Autodesk Inventor part; units mm, degrees
(part 2 of 5)
sketch "Sketch4" plane through (0, 0, 3) normal (0, 0, 1) x (1, 0, 0)
  line L0 (57.5, 215) -> (-78, 215) projected
  line L1 (-78, 215) -> (-78, 46.0635) projected
  line L2 (-78, 46.0635) -> (-75, 46.0635) projected
  line L3 (-75, 46.0635) -> (-75, 40.8932) projected
  line L4 (-75, 40.8932) -> (-78, 40.8932) projected
  line L5 (-78, 40.8932) -> (-78, 30.6062) projected
  line L6 (-78, 30.6062) -> (-75, 30.6062) projected
  line L7 (-75, 30.6062) -> (-75, 20.5478) projected
  line L8 (-75, 20.5478) -> (-78, 20.5478) projected
  line L9 (-78, 20.5478) -> (-78, 10.2608) projected
  line L10 (-78, 10.2608) -> (-75, 10.2608) projected
  line L11 (-75, 10.2608) -> (-75, -0.1068) projected
  line L12 (-75, -0.1068) -> (-78, -0.1068) projected
  line L13 (-78, -0.1068) -> (-78, -10.3938) projected
  line L14 (-78, -10.3938) -> (-75, -10.3938) projected
  line L15 (-75, -10.3938) -> (-75, -20.4522) projected
  line L16 (-75, -20.4522) -> (-78, -20.4522) projected
  line L17 (-78, -20.4522) -> (-78, -30.7392) projected
  line L18 (-78, -30.7392) -> (-75, -30.7392) projected
  line L19 (-75, -30.7392) -> (-75, -41.1068) projected
  line L20 (-75, -41.1068) -> (-78, -41.1068) projected
  line L21 (-78, -41.1068) -> (-78, -51.3938) projected
  line L22 (-78, -51.3938) -> (-75, -51.3938) projected
  line L23 (-75, -51.3938) -> (-75, -61.4522) projected
  line L24 (-75, -61.4522) -> (-78, -61.4522) projected
  line L25 (-78, -61.4522) -> (-78, -71.7392) projected
  line L26 (-78, -71.7392) -> (-75, -71.7392) projected
  line L27 (-75, -71.7392) -> (-75, -82.1068) projected
  line L28 (-75, -82.1068) -> (-78, -82.1068) projected
  line L29 (-78, -82.1068) -> (-78, -92.3938) projected
  line L30 (-78, -92.3938) -> (-75, -92.3938) projected
  line L31 (-75, -92.3938) -> (-75, -102.4522) projected
  line L32 (-75, -102.4522) -> (-78, -102.4522) projected
  line L33 (-78, -102.4522) -> (-78, -130) projected
  line L34 (-78, -130) -> (-55.8933, -130) projected
  line L35 (-55.8933, -130) -> (-55.8933, -135) projected
  line L36 (-55.8933, -135) -> (-25.3933, -135) projected
  line L37 (-25.3933, -135) -> (-25.3933, -147.5) projected
  line L38 (-25.3933, -147.5) -> (23.6067, -147.5) projected
  line L39 (23.6067, -147.5) -> (23.6067, -135) projected
  line L40 (23.6067, -135) -> (54.1067, -135) projected
  line L41 (54.1067, -135) -> (54.1067, -130) projected
  line L42 (54.1067, -130) -> (75, -130) projected
  line L43 (75, -130) -> (75, -111.1237) projected
  arc A0 (75, -111.1237) -> (74, -110.1237) centre (74, -111.1237) ccw projected
  line L44 (74, -110.1237) -> (64.4142, -110.1237) projected
  arc A1 (64.4142, -110.1237) -> (63.7071, -110.4166) centre (64.4142, -111.1237) ccw projected
  line L45 (63.7071, -110.4166) -> (59.2929, -114.8308) projected
  arc A2 (58.5858, -115.1237) -> (59.2929, -114.8308) centre (58.5858, -114.1237) ccw projected
  line L46 (58.5858, -115.1237) -> (43.2196, -115.1237) projected
  arc A3 (42.2196, -114.1237) -> (43.2196, -115.1237) centre (43.2196, -114.1237) ccw projected
  line L47 (42.2196, -114.1237) -> (42.2196, -104.6674) projected
  arc A4 (42.2196, -104.6674) -> (40.773, -102.7455) centre (40.2196, -104.6674) ccw projected
  arc A5 (39.7673, -102.1811) -> (40.773, -102.7455) centre (41.4696, -100.3262) ccw projected
  arc A6 (39.1196, -100.7076) -> (39.7673, -102.1811) centre (41.1196, -100.7076) ccw projected
  line L48 (39.1196, -100.7076) -> (39.1196, -95.7515) projected
  arc A7 (39.7673, -94.2779) -> (39.1196, -95.7515) centre (41.1196, -95.7515) ccw projected
  arc A8 (39.937, -94.1354) -> (39.7673, -94.2779) centre (41.4696, -96.1328) ccw projected
  arc A9 (39.937, -94.1354) -> (40.7196, -92.5486) centre (38.7196, -92.5486) ccw projected
  line L49 (40.7196, -92.5486) -> (40.7196, -83.4104) projected
  arc A10 (40.7196, -83.4104) -> (39.937, -81.8236) centre (38.7196, -83.4104) ccw projected
  arc A11 (39.7673, -81.6811) -> (39.937, -81.8236) centre (41.4696, -79.8262) ccw projected
  arc A12 (39.1196, -80.2076) -> (39.7673, -81.6811) centre (41.1196, -80.2076) ccw projected
  line L50 (39.1196, -80.2076) -> (39.1196, -75.2515) projected
  arc A13 (39.7673, -73.7779) -> (39.1196, -75.2515) centre (41.1196, -75.2515) ccw projected
  arc A14 (39.937, -73.6354) -> (39.7673, -73.7779) centre (41.4696, -75.6328) ccw projected
  arc A15 (39.937, -73.6354) -> (40.7196, -72.0486) centre (38.7196, -72.0486) ccw projected
  line L51 (40.7196, -72.0486) -> (40.7196, -62.9104) projected
  arc A16 (40.7196, -62.9104) -> (39.937, -61.3236) centre (38.7196, -62.9104) ccw projected
  arc A17 (39.7673, -61.1811) -> (39.937, -61.3236) centre (41.4696, -59.3262) ccw projected
  arc A18 (39.1196, -59.7076) -> (39.7673, -61.1811) centre (41.1196, -59.7076) ccw projected
  line L52 (39.1196, -59.7076) -> (39.1196, -54.7515) projected
  arc A19 (39.7673, -53.2779) -> (39.1196, -54.7515) centre (41.1196, -54.7515) ccw projected
  arc A20 (39.937, -53.1354) -> (39.7673, -53.2779) centre (41.4696, -55.1328) ccw projected
  arc A21 (39.937, -53.1354) -> (40.7196, -51.5486) centre (38.7196, -51.5486) ccw projected
  line L53 (40.7196, -51.5486) -> (40.7196, -42.4104) projected
  arc A22 (40.7196, -42.4104) -> (39.937, -40.8236) centre (38.7196, -42.4104) ccw projected
  arc A23 (39.7673, -40.6811) -> (39.937, -40.8236) centre (41.4696, -38.8262) ccw projected
  arc A24 (39.1196, -39.2076) -> (39.7673, -40.6811) centre (41.1196, -39.2076) ccw projected
  line L54 (39.1196, -39.2076) -> (39.1196, -34.2515) projected
  arc A25 (39.7673, -32.7779) -> (39.1196, -34.2515) centre (41.1196, -34.2515) ccw projected
  arc A26 (39.937, -32.6354) -> (39.7673, -32.7779) centre (41.4696, -34.6328) ccw projected
  arc A27 (39.937, -32.6354) -> (40.7196, -31.0486) centre (38.7196, -31.0486) ccw projected
  line L55 (40.7196, -31.0486) -> (40.7196, -21.9104) projected
  arc A28 (40.7196, -21.9104) -> (39.937, -20.3236) centre (38.7196, -21.9104) ccw projected
  arc A29 (39.7673, -20.1811) -> (39.937, -20.3236) centre (41.4696, -18.3262) ccw projected
  arc A30 (39.1196, -18.7076) -> (39.7673, -20.1811) centre (41.1196, -18.7076) ccw projected
  line L56 (39.1196, -18.7076) -> (39.1196, -13.7515) projected
  arc A31 (39.7673, -12.2779) -> (39.1196, -13.7515) centre (41.1196, -13.7515) ccw projected
  arc A32 (39.937, -12.1354) -> (39.7673, -12.2779) centre (41.4696, -14.1328) ccw projected
  arc A33 (39.937, -12.1354) -> (40.7196, -10.5486) centre (38.7196, -10.5486) ccw projected
  line L57 (40.7196, -10.5486) -> (40.7196, -1.4104) projected
  arc A34 (40.7196, -1.4104) -> (39.937, 0.1764) centre (38.7196, -1.4104) ccw projected
  arc A35 (39.7673, 0.3189) -> (39.937, 0.1764) centre (41.4696, 2.1738) ccw projected
  arc A36 (39.1196, 1.7924) -> (39.7673, 0.3189) centre (41.1196, 1.7924) ccw projected
  line L58 (39.1196, 1.7924) -> (39.1196, 6.7485) projected
  arc A37 (39.7673, 8.2221) -> (39.1196, 6.7485) centre (41.1196, 6.7485) ccw projected
  arc A38 (39.937, 8.3646) -> (39.7673, 8.2221) centre (41.4696, 6.3672) ccw projected
  arc A39 (39.937, 8.3646) -> (40.7196, 9.9514) centre (38.7196, 9.9514) ccw projected
  line L59 (40.7196, 9.9514) -> (40.7196, 19.0896) projected
  arc A40 (40.7196, 19.0896) -> (39.937, 20.6764) centre (38.7196, 19.0896) ccw projected
  arc A41 (39.7673, 20.8189) -> (39.937, 20.6764) centre (41.4696, 22.6738) ccw projected
  arc A42 (39.1196, 22.2924) -> (39.7673, 20.8189) centre (41.1196, 22.2924) ccw projected
  line L60 (39.1196, 22.2924) -> (39.1196, 27.2485) projected
  arc A43 (39.7673, 28.7221) -> (39.1196, 27.2485) centre (41.1196, 27.2485) ccw projected
  arc A44 (39.937, 28.8646) -> (39.7673, 28.7221) centre (41.4696, 26.8672) ccw projected
  arc A45 (39.937, 28.8646) -> (40.7196, 30.4514) centre (38.7196, 30.4514) ccw projected
  line L61 (40.7196, 30.4514) -> (40.7196, 39.5896) projected
  arc A46 (40.7196, 39.5896) -> (39.937, 41.1764) centre (38.7196, 39.5896) ccw projected
  arc A47 (39.7673, 41.3189) -> (39.937, 41.1764) centre (41.4696, 43.1738) ccw projected
  arc A48 (39.1196, 42.7924) -> (39.7673, 41.3189) centre (41.1196, 42.7924) ccw projected
  line L62 (39.1196, 42.7924) -> (39.1196, 47.7485) projected
  arc A49 (39.7673, 49.2221) -> (39.1196, 47.7485) centre (41.1196, 47.7485) ccw projected
  arc A50 (43.3362, 49.0566) -> (39.7673, 49.2221) centre (41.4696, 47.3672) ccw projected
  arc A51 (43.3362, 49.0566) -> (44.819, 48.3987) centre (44.819, 50.3987) ccw projected
  line L63 (44.819, 48.3987) -> (75, 48.3987) projected
  line L64 (75, 48.3987) -> (75, 184.5) projected
  line L65 (75, 184.5) -> (57.5, 184.5) projected
  line L66 (57.5, 184.5) -> (57.5, 215) projected
  line L67 (-69.3194, 50.0635) -> (-69.3194, 207.0635) projected
  arc A52 (-68.3194, 208.0635) -> (-69.3194, 207.0635) centre (-68.3194, 207.0635) ccw projected
  line L68 (-68.3194, 208.0635) -> (-25.6194, 208.0635) projected
  arc A53 (-24.6194, 207.0635) -> (-25.6194, 208.0635) centre (-25.6194, 207.0635) ccw projected
  line L69 (-24.6194, 207.0635) -> (-24.6194, 50.0635) projected
  arc A54 (-25.6194, 49.0635) -> (-24.6194, 50.0635) centre (-25.6194, 50.0635) ccw projected
  line L70 (-25.6194, 49.0635) -> (-68.3194, 49.0635) projected
  arc A55 (-69.3194, 50.0635) -> (-68.3194, 49.0635) centre (-68.3194, 50.0635) ccw projected
  arc A56 (-6.9692, 137.8876) -> (4.019, 134.5987) centre (4.019, 154.5987) ccw projected
  arc A57 (-13.8416, 143.5179) -> (-6.9692, 137.8876) centre (16.3806, 173.3987) ccw projected
  arc A58 (-19.6194, 157.5794) -> (-13.8416, 143.5179) centre (0.3806, 157.5794) ccw projected
  line L71 (-19.6194, 157.5794) -> (-19.6194, 189.218) projected
  arc A59 (-13.8416, 203.2796) -> (-19.6194, 189.218) centre (0.3806, 189.218) ccw projected
  arc A60 (-6.9692, 208.9099) -> (-13.8416, 203.2796) centre (16.3806, 173.3987) ccw projected
  arc A61 (4.019, 212.1987) -> (-6.9692, 208.9099) centre (4.019, 192.1987) ccw projected
  line L72 (4.019, 212.1987) -> (28.7422, 212.1987) projected
  arc A62 (39.7304, 208.9099) -> (28.7422, 212.1987) centre (28.7422, 192.1987) ccw projected
  arc A63 (46.6028, 203.2796) -> (39.7304, 208.9099) centre (16.3806, 173.3987) ccw projected
  arc A64 (52.3806, 189.218) -> (46.6028, 203.2796) centre (32.3806, 189.218) ccw projected
  line L73 (52.3806, 189.218) -> (52.3806, 157.5794) projected
  arc A65 (46.6028, 143.5179) -> (52.3806, 157.5794) centre (32.3806, 157.5794) ccw projected
  arc A66 (39.7304, 137.8876) -> (46.6028, 143.5179) centre (16.3806, 173.3987) ccw projected
  arc A67 (28.7422, 134.5987) -> (39.7304, 137.8876) centre (28.7422, 154.5987) ccw projected
  line L74 (28.7422, 134.5987) -> (4.019, 134.5987) projected
  arc A68 (-6.9692, 54.8876) -> (4.019, 51.5987) centre (4.019, 71.5987) ccw projected
  arc A69 (-13.8416, 60.5179) -> (-6.9692, 54.8876) centre (16.3806, 90.3987) ccw projected
  arc A70 (-19.6194, 74.5794) -> (-13.8416, 60.5179) centre (0.3806, 74.5794) ccw projected
  line L75 (-19.6194, 74.5794) -> (-19.6194, 106.218) projected
  arc A71 (-13.8416, 120.2796) -> (-19.6194, 106.218) centre (0.3806, 106.218) ccw projected
  arc A72 (-6.9692, 125.9099) -> (-13.8416, 120.2796) centre (16.3806, 90.3987) ccw projected
  arc A73 (4.019, 129.1987) -> (-6.9692, 125.9099) centre (4.019, 109.1987) ccw projected
  line L76 (4.019, 129.1987) -> (28.7422, 129.1987) projected
  arc A74 (39.7304, 125.9099) -> (28.7422, 129.1987) centre (28.7422, 109.1987) ccw projected
  arc A75 (46.6028, 120.2796) -> (39.7304, 125.9099) centre (16.3806, 90.3987) ccw projected
  arc A76 (52.3806, 106.218) -> (46.6028, 120.2796) centre (32.3806, 106.218) ccw projected
  line L77 (52.3806, 106.218) -> (52.3806, 74.5794) projected
  arc A77 (46.6028, 60.5179) -> (52.3806, 74.5794) centre (32.3806, 74.5794) ccw projected
  arc A78 (39.7304, 54.8876) -> (46.6028, 60.5179) centre (16.3806, 90.3987) ccw projected
  arc A79 (28.7422, 51.5987) -> (39.7304, 54.8876) centre (28.7422, 71.5987) ccw projected
  line L78 (28.7422, 51.5987) -> (4.019, 51.5987) projected
  arc A80 (31.7396, -114.6081) -> (34.7396, -111.6081) centre (31.7396, -111.6081) ccw projected
  line L79 (31.7396, -114.6081) -> (-55.9404, -114.6081) projected
  arc A81 (-58.9404, -111.6081) -> (-55.9404, -114.6081) centre (-55.9404, -111.6081) ccw projected
  line L80 (-58.9404, -111.6081) -> (-58.9404, -101.7281) projected
  arc A82 (-55.9404, -98.7281) -> (-58.9404, -101.7281) centre (-55.9404, -101.7281) ccw projected
  line L81 (-55.9404, -98.7281) -> (31.7396, -98.7281) projected
  arc A83 (34.7396, -101.7281) -> (31.7396, -98.7281) centre (31.7396, -101.7281) ccw projected
  line L82 (34.7396, -101.7281) -> (34.7396, -111.6081) projected
  arc A84 (34.7396, -81.3827) -> (31.7396, -78.3827) centre (31.7396, -81.3827) ccw projected
  line L83 (34.7396, -81.3827) -> (34.7396, -91.2627) projected
  arc A85 (31.7396, -94.2627) -> (34.7396, -91.2627) centre (31.7396, -91.2627) ccw projected
  line L84 (31.7396, -94.2627) -> (-55.9404, -94.2627) projected
  arc A86 (-58.9404, -91.2627) -> (-55.9404, -94.2627) centre (-55.9404, -91.2627) ccw projected
  line L85 (-58.9404, -91.2627) -> (-58.9404, -81.3827) projected
  arc A87 (-55.9404, -78.3827) -> (-58.9404, -81.3827) centre (-55.9404, -81.3827) ccw projected
  line L86 (-55.9404, -78.3827) -> (31.7396, -78.3827) projected
  line L87 (31.7396, -33.2265) -> (-55.9404, -33.2265) projected
  arc A88 (-58.9404, -30.2265) -> (-55.9404, -33.2265) centre (-55.9404, -30.2265) ccw projected
  line L88 (-58.9404, -30.2265) -> (-58.9404, -20.3465) projected
  arc A89 (-55.9404, -17.3465) -> (-58.9404, -20.3465) centre (-55.9404, -20.3465) ccw projected
  line L89 (-55.9404, -17.3465) -> (31.7396, -17.3465) projected
  arc A90 (34.7396, -20.3465) -> (31.7396, -17.3465) centre (31.7396, -20.3465) ccw projected
  line L90 (34.7396, -20.3465) -> (34.7396, -30.2265) projected
  arc A91 (31.7396, -33.2265) -> (34.7396, -30.2265) centre (31.7396, -30.2265) ccw projected
  line L91 (-55.9404, -58.0373) -> (31.7396, -58.0373) projected
  arc A92 (34.7396, -61.0373) -> (31.7396, -58.0373) centre (31.7396, -61.0373) ccw projected
  line L92 (34.7396, -61.0373) -> (34.7396, -70.9173) projected
  arc A93 (31.7396, -73.9173) -> (34.7396, -70.9173) centre (31.7396, -70.9173) ccw projected
  line L93 (31.7396, -73.9173) -> (-55.9404, -73.9173) projected
  arc A94 (-58.9404, -70.9173) -> (-55.9404, -73.9173) centre (-55.9404, -70.9173) ccw projected
  line L94 (-58.9404, -70.9173) -> (-58.9404, -61.0373) projected
  arc A95 (-55.9404, -58.0373) -> (-58.9404, -61.0373) centre (-55.9404, -61.0373) ccw projected
  arc A96 (-55.9404, -37.6919) -> (-58.9404, -40.6919) centre (-55.9404, -40.6919) ccw projected
  line L95 (-55.9404, -37.6919) -> (31.7396, -37.6919) projected
  arc A97 (34.7396, -40.6919) -> (31.7396, -37.6919) centre (31.7396, -40.6919) ccw projected
  line L96 (34.7396, -40.6919) -> (34.7396, -50.5719) projected
  arc A98 (31.7396, -53.5719) -> (34.7396, -50.5719) centre (31.7396, -50.5719) ccw projected
  line L97 (31.7396, -53.5719) -> (-55.9404, -53.5719) projected
  arc A99 (-58.9404, -50.5719) -> (-55.9404, -53.5719) centre (-55.9404, -50.5719) ccw projected
  line L98 (-58.9404, -50.5719) -> (-58.9404, -40.6919) projected
  arc A100 (-55.9404, 2.9989) -> (-58.9404, -0.0011) centre (-55.9404, -0.0011) ccw projected
  line L99 (-55.9404, 2.9989) -> (31.7396, 2.9989) projected
  arc A101 (34.7396, -0.0011) -> (31.7396, 2.9989) centre (31.7396, -0.0011) ccw projected
  line L100 (34.7396, -0.0011) -> (34.7396, -9.8811) projected
  arc A102 (31.7396, -12.8811) -> (34.7396, -9.8811) centre (31.7396, -9.8811) ccw projected
  line L101 (31.7396, -12.8811) -> (-55.9404, -12.8811) projected
  arc A103 (-58.9404, -9.8811) -> (-55.9404, -12.8811) centre (-55.9404, -9.8811) ccw projected
  line L102 (-58.9404, -9.8811) -> (-58.9404, -0.0011) projected
  line L103 (-58.9404, 30.8097) -> (-58.9404, 40.6897) projected
  arc A104 (-55.9404, 43.6897) -> (-58.9404, 40.6897) centre (-55.9404, 40.6897) ccw projected
  line L104 (-55.9404, 43.6897) -> (31.7396, 43.6897) projected
  arc A105 (34.7396, 40.6897) -> (31.7396, 43.6897) centre (31.7396, 40.6897) ccw projected
  line L105 (34.7396, 40.6897) -> (34.7396, 30.8097) projected
  arc A106 (31.7396, 27.8097) -> (34.7396, 30.8097) centre (31.7396, 30.8097) ccw projected
  line L106 (31.7396, 27.8097) -> (-55.9404, 27.8097) projected
  arc A107 (-58.9404, 30.8097) -> (-55.9404, 27.8097) centre (-55.9404, 30.8097) ccw projected
  line L107 (-58.9404, 10.4643) -> (-58.9404, 20.3443) projected
  arc A108 (-55.9404, 23.3443) -> (-58.9404, 20.3443) centre (-55.9404, 20.3443) ccw projected
  line L108 (-55.9404, 23.3443) -> (31.7396, 23.3443) projected
  arc A109 (34.7396, 20.3443) -> (31.7396, 23.3443) centre (31.7396, 20.3443) ccw projected
  line L109 (34.7396, 20.3443) -> (34.7396, 10.4643) projected
  arc A110 (31.7396, 7.4643) -> (34.7396, 10.4643) centre (31.7396, 10.4643) ccw projected
  line L110 (31.7396, 7.4643) -> (-55.9404, 7.4643) projected
  arc A111 (-58.9404, 10.4643) -> (-55.9404, 7.4643) centre (-55.9404, 10.4643) ccw projected
  circle A112 centre (16.1067, -140) radius 2.25 projected
  circle A113 centre (-17.8933, -140) radius 2.25 projected
  circle A114 centre (65, -117.6237) radius 2.25 projected
  circle A115 centre (65, 174.5) radius 2.25 projected
  circle A116 centre (65, 131.8987) radius 2.25 projected
  circle A117 centre (65, 58.3987) radius 2.25 projected
  circle A118 centre (-19.3694, 54.6487) radius 1.2 projected
  circle A119 centre (-19.3694, 209.1487) radius 1.2 projected
  circle A120 centre (-19.3694, 137.6487) radius 1.2 projected
  circle A121 centre (52.1306, 54.6487) radius 1.2 projected
  circle A122 centre (52.1306, 209.1487) radius 1.2 projected
  circle A123 centre (52.1306, 137.6487) radius 1.2 projected
  circle A124 centre (52.1306, 126.1487) radius 1.2 projected
  circle A125 centre (-19.3694, 126.1487) radius 1.2 projected
  line L111 (-78, -102.4522) -> (-78, -130) projected
  line L112 (-78, -112.7392) -> (-75, -112.7392)
  line L113 (-75, -112.7392) -> (-75, -130)
  line L114 (-78, -130) -> (-55.8933, -130) projected
  line L115 (54.1067, -135) -> (54.1067, -130) projected
  line L116 (54.1067, -130) -> (-55.8933, -130)
  line L117 (-25.3933, -135) -> (-25.3933, -130)
  line L118 (23.6067, -135) -> (23.6067, -130)
  line L119 (23.6067, -147.5) -> (23.6067, -135) projected
  line L120 (23.6067, -135) -> (54.1067, -135)
  line L121 (54.1067, -135) -> (54.1067, -130)
  line L122 (54.1067, -130) -> (23.6067, -130)
  line L123 (23.6067, -130) -> (23.6067, -135)
  line L124 (-55.8933, -135) -> (-25.3933, -135) projected
  line L125 (-25.3933, -135) -> (-55.8933, -135)
  line L126 (-55.8933, -135) -> (-55.8933, -130)
  line L127 (-55.8933, -130) -> (-25.3933, -130)
  line L128 (-25.3933, -130) -> (-25.3933, -135)
  line L129 (-78, -130) -> (-75, -130)
  line L130 (-75, -130) -> (-75, -112.7392)
  line L131 (-75, -112.7392) -> (-78, -112.7392)
  line L132 (-78, -112.7392) -> (-78, -130)
  point P0 (0, 0)
  dimension "d40" = 10.287
  dimension "d41" = 3
  dimension "d42" = 3
  dimension "d43" = 10.287
  constraints: 34 end point, 7 perpendicular, 6 parallel, 4 horizontal, 4 point on line
  measures "d40" distance of L28.end L29.end
  measures "d41" distance of L31.end L32.end
  measures "d42" distance of L112.start L112.end
  measures "d43" distance between parallel lines of L32 L112
extrude "Extrusion4" cut sketch "Sketch4" against normal blind 10 contours L112 L113 L34 L33 | L116 L117 L36 L35 | L116 L41 L40 L118
sketch "Sketch5" plane through (0, 0, 3) normal (0, 0, 1) x (1, 0, 0)
  circle A0 centre (-19.3694, 126.1487) radius 1.2 projected
  circle A1 centre (52.1306, 126.1487) radius 1.2 projected
  circle A2 centre (52.1306, 137.6487) radius 1.2 projected
  circle A3 centre (52.1306, 209.1487) radius 1.2 projected
  circle A4 centre (52.1306, 54.6487) radius 1.2 projected
  circle A5 centre (-19.3694, 137.6487) radius 1.2 projected
  circle A6 centre (-19.3694, 209.1487) radius 1.2 projected
  circle A7 centre (-19.3694, 54.6487) radius 1.2 projected
  circle A8 centre (65, 58.3987) radius 2.25 projected
  circle A9 centre (65, 131.8987) radius 2.25 projected
  circle A10 centre (65, 174.5) radius 2.25 projected
  circle A11 centre (65, -117.6237) radius 2.25 projected
  circle A12 centre (-17.8933, -140) radius 2.25 projected
  circle A13 centre (16.1067, -140) radius 2.25 projected
  line L0 (-58.9404, 10.4643) -> (-58.9404, 20.3443) projected
  arc A14 (-55.9404, 23.3443) -> (-58.9404, 20.3443) centre (-55.9404, 20.3443) ccw projected
  line L1 (-55.9404, 23.3443) -> (31.7396, 23.3443) projected
  arc A15 (34.7396, 20.3443) -> (31.7396, 23.3443) centre (31.7396, 20.3443) ccw projected
  line L2 (34.7396, 20.3443) -> (34.7396, 10.4643) projected
  arc A16 (31.7396, 7.4643) -> (34.7396, 10.4643) centre (31.7396, 10.4643) ccw projected
  line L3 (31.7396, 7.4643) -> (-55.9404, 7.4643) projected
  arc A17 (-58.9404, 10.4643) -> (-55.9404, 7.4643) centre (-55.9404, 10.4643) ccw projected
  line L4 (-58.9404, 30.8097) -> (-58.9404, 40.6897) projected
  arc A18 (-55.9404, 43.6897) -> (-58.9404, 40.6897) centre (-55.9404, 40.6897) ccw projected
  line L5 (-55.9404, 43.6897) -> (31.7396, 43.6897) projected
  arc A19 (34.7396, 40.6897) -> (31.7396, 43.6897) centre (31.7396, 40.6897) ccw projected
  line L6 (34.7396, 40.6897) -> (34.7396, 30.8097) projected
  arc A20 (31.7396, 27.8097) -> (34.7396, 30.8097) centre (31.7396, 30.8097) ccw projected
  line L7 (31.7396, 27.8097) -> (-55.9404, 27.8097) projected
  arc A21 (-58.9404, 30.8097) -> (-55.9404, 27.8097) centre (-55.9404, 30.8097) ccw projected
  arc A22 (-55.9404, 2.9989) -> (-58.9404, -0.0011) centre (-55.9404, -0.0011) ccw projected
  line L8 (-55.9404, 2.9989) -> (31.7396, 2.9989) projected
  arc A23 (34.7396, -0.0011) -> (31.7396, 2.9989) centre (31.7396, -0.0011) ccw projected
  line L9 (34.7396, -0.0011) -> (34.7396, -9.8811) projected
  arc A24 (31.7396, -12.8811) -> (34.7396, -9.8811) centre (31.7396, -9.8811) ccw projected
  line L10 (31.7396, -12.8811) -> (-55.9404, -12.8811) projected
  arc A25 (-58.9404, -9.8811) -> (-55.9404, -12.8811) centre (-55.9404, -9.8811) ccw projected
  line L11 (-58.9404, -9.8811) -> (-58.9404, -0.0011) projected
  arc A26 (-55.9404, -37.6919) -> (-58.9404, -40.6919) centre (-55.9404, -40.6919) ccw projected
  line L12 (-55.9404, -37.6919) -> (31.7396, -37.6919) projected
  arc A27 (34.7396, -40.6919) -> (31.7396, -37.6919) centre (31.7396, -40.6919) ccw projected
  line L13 (34.7396, -40.6919) -> (34.7396, -50.5719) projected
  arc A28 (31.7396, -53.5719) -> (34.7396, -50.5719) centre (31.7396, -50.5719) ccw projected
  line L14 (31.7396, -53.5719) -> (-55.9404, -53.5719) projected
  arc A29 (-58.9404, -50.5719) -> (-55.9404, -53.5719) centre (-55.9404, -50.5719) ccw projected
  line L15 (-58.9404, -50.5719) -> (-58.9404, -40.6919) projected
  line L16 (-55.9404, -58.0373) -> (31.7396, -58.0373) projected
  arc A30 (34.7396, -61.0373) -> (31.7396, -58.0373) centre (31.7396, -61.0373) ccw projected
  line L17 (34.7396, -61.0373) -> (34.7396, -70.9173) projected
  arc A31 (31.7396, -73.9173) -> (34.7396, -70.9173) centre (31.7396, -70.9173) ccw projected
  line L18 (31.7396, -73.9173) -> (-55.9404, -73.9173) projected
  arc A32 (-58.9404, -70.9173) -> (-55.9404, -73.9173) centre (-55.9404, -70.9173) ccw projected
  line L19 (-58.9404, -70.9173) -> (-58.9404, -61.0373) projected
  arc A33 (-55.9404, -58.0373) -> (-58.9404, -61.0373) centre (-55.9404, -61.0373) ccw projected
  line L20 (31.7396, -33.2265) -> (-55.9404, -33.2265) projected
  arc A34 (-58.9404, -30.2265) -> (-55.9404, -33.2265) centre (-55.9404, -30.2265) ccw projected
  line L21 (-58.9404, -30.2265) -> (-58.9404, -20.3465) projected
  arc A35 (-55.9404, -17.3465) -> (-58.9404, -20.3465) centre (-55.9404, -20.3465) ccw projected
  line L22 (-55.9404, -17.3465) -> (31.7396, -17.3465) projected
  arc A36 (34.7396, -20.3465) -> (31.7396, -17.3465) centre (31.7396, -20.3465) ccw projected
  line L23 (34.7396, -20.3465) -> (34.7396, -30.2265) projected
  arc A37 (31.7396, -33.2265) -> (34.7396, -30.2265) centre (31.7396, -30.2265) ccw projected
  arc A38 (34.7396, -81.3827) -> (31.7396, -78.3827) centre (31.7396, -81.3827) ccw projected
  line L24 (34.7396, -81.3827) -> (34.7396, -91.2627) projected
  arc A39 (31.7396, -94.2627) -> (34.7396, -91.2627) centre (31.7396, -91.2627) ccw projected
  line L25 (31.7396, -94.2627) -> (-55.9404, -94.2627) projected
  arc A40 (-58.9404, -91.2627) -> (-55.9404, -94.2627) centre (-55.9404, -91.2627) ccw projected
  line L26 (-58.9404, -91.2627) -> (-58.9404, -81.3827) projected
  arc A41 (-55.9404, -78.3827) -> (-58.9404, -81.3827) centre (-55.9404, -81.3827) ccw projected
  line L27 (-55.9404, -78.3827) -> (31.7396, -78.3827) projected
  arc A42 (31.7396, -114.6081) -> (34.7396, -111.6081) centre (31.7396, -111.6081) ccw projected
  line L28 (31.7396, -114.6081) -> (-55.9404, -114.6081) projected
  arc A43 (-58.9404, -111.6081) -> (-55.9404, -114.6081) centre (-55.9404, -111.6081) ccw projected
  line L29 (-58.9404, -111.6081) -> (-58.9404, -101.7281) projected
  arc A44 (-55.9404, -98.7281) -> (-58.9404, -101.7281) centre (-55.9404, -101.7281) ccw projected
  line L30 (-55.9404, -98.7281) -> (31.7396, -98.7281) projected
  arc A45 (34.7396, -101.7281) -> (31.7396, -98.7281) centre (31.7396, -101.7281) ccw projected
  line L31 (34.7396, -101.7281) -> (34.7396, -111.6081) projected
  arc A46 (-6.9692, 54.8876) -> (4.019, 51.5987) centre (4.019, 71.5987) ccw projected
  arc A47 (-13.8416, 60.5179) -> (-6.9692, 54.8876) centre (16.3806, 90.3987) ccw projected
  arc A48 (-19.6194, 74.5794) -> (-13.8416, 60.5179) centre (0.3806, 74.5794) ccw projected
  line L32 (-19.6194, 74.5794) -> (-19.6194, 106.218) projected
  arc A49 (-13.8416, 120.2796) -> (-19.6194, 106.218) centre (0.3806, 106.218) ccw projected
  arc A50 (-6.9692, 125.9099) -> (-13.8416, 120.2796) centre (16.3806, 90.3987) ccw projected
  arc A51 (4.019, 129.1987) -> (-6.9692, 125.9099) centre (4.019, 109.1987) ccw projected
  line L33 (4.019, 129.1987) -> (28.7422, 129.1987) projected
  arc A52 (39.7304, 125.9099) -> (28.7422, 129.1987) centre (28.7422, 109.1987) ccw projected
  arc A53 (46.6028, 120.2796) -> (39.7304, 125.9099) centre (16.3806, 90.3987) ccw projected
  arc A54 (52.3806, 106.218) -> (46.6028, 120.2796) centre (32.3806, 106.218) ccw projected
  line L34 (52.3806, 106.218) -> (52.3806, 74.5794) projected
  arc A55 (46.6028, 60.5179) -> (52.3806, 74.5794) centre (32.3806, 74.5794) ccw projected
  arc A56 (39.7304, 54.8876) -> (46.6028, 60.5179) centre (16.3806, 90.3987) ccw projected
  arc A57 (28.7422, 51.5987) -> (39.7304, 54.8876) centre (28.7422, 71.5987) ccw projected
  line L35 (28.7422, 51.5987) -> (4.019, 51.5987) projected
  arc A58 (-6.9692, 137.8876) -> (4.019, 134.5987) centre (4.019, 154.5987) ccw projected
  arc A59 (-13.8416, 143.5179) -> (-6.9692, 137.8876) centre (16.3806, 173.3987) ccw projected
  arc A60 (-19.6194, 157.5794) -> (-13.8416, 143.5179) centre (0.3806, 157.5794) ccw projected
  line L36 (-19.6194, 157.5794) -> (-19.6194, 189.218) projected
  arc A61 (-13.8416, 203.2796) -> (-19.6194, 189.218) centre (0.3806, 189.218) ccw projected
  arc A62 (-6.9692, 208.9099) -> (-13.8416, 203.2796) centre (16.3806, 173.3987) ccw projected
  arc A63 (4.019, 212.1987) -> (-6.9692, 208.9099) centre (4.019, 192.1987) ccw projected
  line L37 (4.019, 212.1987) -> (28.7422, 212.1987) projected
  arc A64 (39.7304, 208.9099) -> (28.7422, 212.1987) centre (28.7422, 192.1987) ccw projected
  arc A65 (46.6028, 203.2796) -> (39.7304, 208.9099) centre (16.3806, 173.3987) ccw projected
  arc A66 (52.3806, 189.218) -> (46.6028, 203.2796) centre (32.3806, 189.218) ccw projected
  line L38 (52.3806, 189.218) -> (52.3806, 157.5794) projected
  arc A67 (46.6028, 143.5179) -> (52.3806, 157.5794) centre (32.3806, 157.5794) ccw projected
  arc A68 (39.7304, 137.8876) -> (46.6028, 143.5179) centre (16.3806, 173.3987) ccw projected
  arc A69 (28.7422, 134.5987) -> (39.7304, 137.8876) centre (28.7422, 154.5987) ccw projected
  line L39 (28.7422, 134.5987) -> (4.019, 134.5987) projected
  line L40 (-69.3194, 50.0635) -> (-69.3194, 207.0635) projected
  arc A70 (-68.3194, 208.0635) -> (-69.3194, 207.0635) centre (-68.3194, 207.0635) ccw projected
  line L41 (-68.3194, 208.0635) -> (-25.6194, 208.0635) projected
  arc A71 (-24.6194, 207.0635) -> (-25.6194, 208.0635) centre (-25.6194, 207.0635) ccw projected
  line L42 (-24.6194, 207.0635) -> (-24.6194, 50.0635) projected
  arc A72 (-25.6194, 49.0635) -> (-24.6194, 50.0635) centre (-25.6194, 50.0635) ccw projected
  line L43 (-25.6194, 49.0635) -> (-68.3194, 49.0635) projected
  arc A73 (-69.3194, 50.0635) -> (-68.3194, 49.0635) centre (-68.3194, 50.0635) ccw projected
  line L44 (23.6067, -147.5) -> (23.6067, -130) projected
  line L45 (23.6067, -130) -> (75, -130) projected
  line L46 (75, -130) -> (75, -111.1237) projected
  arc A74 (75, -111.1237) -> (74, -110.1237) centre (74, -111.1237) ccw projected
  line L47 (74, -110.1237) -> (64.4142, -110.1237) projected
  arc A75 (64.4142, -110.1237) -> (63.7071, -110.4166) centre (64.4142, -111.1237) ccw projected
  line L48 (63.7071, -110.4166) -> (59.2929, -114.8308) projected
  arc A76 (58.5858, -115.1237) -> (59.2929, -114.8308) centre (58.5858, -114.1237) ccw projected
  line L49 (58.5858, -115.1237) -> (43.2196, -115.1237) projected
  arc A77 (42.2196, -114.1237) -> (43.2196, -115.1237) centre (43.2196, -114.1237) ccw projected
  line L50 (42.2196, -114.1237) -> (42.2196, -104.6674) projected
  arc A78 (42.2196, -104.6674) -> (40.773, -102.7455) centre (40.2196, -104.6674) ccw projected
  arc A79 (39.7673, -102.1811) -> (40.773, -102.7455) centre (41.4696, -100.3262) ccw projected
  arc A80 (39.1196, -100.7076) -> (39.7673, -102.1811) centre (41.1196, -100.7076) ccw projected
  line L51 (39.1196, -100.7076) -> (39.1196, -95.7515) projected
  arc A81 (39.7673, -94.2779) -> (39.1196, -95.7515) centre (41.1196, -95.7515) ccw projected
  arc A82 (39.937, -94.1354) -> (39.7673, -94.2779) centre (41.4696, -96.1328) ccw projected
  arc A83 (39.937, -94.1354) -> (40.7196, -92.5486) centre (38.7196, -92.5486) ccw projected
  line L52 (40.7196, -92.5486) -> (40.7196, -83.4104) projected
  arc A84 (40.7196, -83.4104) -> (39.937, -81.8236) centre (38.7196, -83.4104) ccw projected
  arc A85 (39.7673, -81.6811) -> (39.937, -81.8236) centre (41.4696, -79.8262) ccw projected
  arc A86 (39.1196, -80.2076) -> (39.7673, -81.6811) centre (41.1196, -80.2076) ccw projected
  line L53 (39.1196, -80.2076) -> (39.1196, -75.2515) projected
  arc A87 (39.7673, -73.7779) -> (39.1196, -75.2515) centre (41.1196, -75.2515) ccw projected
  arc A88 (39.937, -73.6354) -> (39.7673, -73.7779) centre (41.4696, -75.6328) ccw projected
  arc A89 (39.937, -73.6354) -> (40.7196, -72.0486) centre (38.7196, -72.0486) ccw projected
  line L54 (40.7196, -72.0486) -> (40.7196, -62.9104) projected
  arc A90 (40.7196, -62.9104) -> (39.937, -61.3236) centre (38.7196, -62.9104) ccw projected
  arc A91 (39.7673, -61.1811) -> (39.937, -61.3236) centre (41.4696, -59.3262) ccw projected
  arc A92 (39.1196, -59.7076) -> (39.7673, -61.1811) centre (41.1196, -59.7076) ccw projected
  line L55 (39.1196, -59.7076) -> (39.1196, -54.7515) projected
  arc A93 (39.7673, -53.2779) -> (39.1196, -54.7515) centre (41.1196, -54.7515) ccw projected
  arc A94 (39.937, -53.1354) -> (39.7673, -53.2779) centre (41.4696, -55.1328) ccw projected
  arc A95 (39.937, -53.1354) -> (40.7196, -51.5486) centre (38.7196, -51.5486) ccw projected
  line L56 (40.7196, -51.5486) -> (40.7196, -42.4104) projected
  arc A96 (40.7196, -42.4104) -> (39.937, -40.8236) centre (38.7196, -42.4104) ccw projected
  arc A97 (39.7673, -40.6811) -> (39.937, -40.8236) centre (41.4696, -38.8262) ccw projected
  arc A98 (39.1196, -39.2076) -> (39.7673, -40.6811) centre (41.1196, -39.2076) ccw projected
  line L57 (39.1196, -39.2076) -> (39.1196, -34.2515) projected
  arc A99 (39.7673, -32.7779) -> (39.1196, -34.2515) centre (41.1196, -34.2515) ccw projected
  arc A100 (39.937, -32.6354) -> (39.7673, -32.7779) centre (41.4696, -34.6328) ccw projected
  arc A101 (39.937, -32.6354) -> (40.7196, -31.0486) centre (38.7196, -31.0486) ccw projected
  line L58 (40.7196, -31.0486) -> (40.7196, -21.9104) projected
  arc A102 (40.7196, -21.9104) -> (39.937, -20.3236) centre (38.7196, -21.9104) ccw projected
  arc A103 (39.7673, -20.1811) -> (39.937, -20.3236) centre (41.4696, -18.3262) ccw projected
  arc A104 (39.1196, -18.7076) -> (39.7673, -20.1811) centre (41.1196, -18.7076) ccw projected
  line L59 (39.1196, -18.7076) -> (39.1196, -13.7515) projected
  arc A105 (39.7673, -12.2779) -> (39.1196, -13.7515) centre (41.1196, -13.7515) ccw projected
  arc A106 (39.937, -12.1354) -> (39.7673, -12.2779) centre (41.4696, -14.1328) ccw projected
  arc A107 (39.937, -12.1354) -> (40.7196, -10.5486) centre (38.7196, -10.5486) ccw projected
  line L60 (40.7196, -10.5486) -> (40.7196, -1.4104) projected
  arc A108 (40.7196, -1.4104) -> (39.937, 0.1764) centre (38.7196, -1.4104) ccw projected
  arc A109 (39.7673, 0.3189) -> (39.937, 0.1764) centre (41.4696, 2.1738) ccw projected
  arc A110 (39.1196, 1.7924) -> (39.7673, 0.3189) centre (41.1196, 1.7924) ccw projected
  line L61 (39.1196, 1.7924) -> (39.1196, 6.7485) projected
  arc A111 (39.7673, 8.2221) -> (39.1196, 6.7485) centre (41.1196, 6.7485) ccw projected
  arc A112 (39.937, 8.3646) -> (39.7673, 8.2221) centre (41.4696, 6.3672) ccw projected
  arc A113 (39.937, 8.3646) -> (40.7196, 9.9514) centre (38.7196, 9.9514) ccw projected
  line L62 (40.7196, 9.9514) -> (40.7196, 19.0896) projected
  arc A114 (40.7196, 19.0896) -> (39.937, 20.6764) centre (38.7196, 19.0896) ccw projected
  arc A115 (39.7673, 20.8189) -> (39.937, 20.6764) centre (41.4696, 22.6738) ccw projected
  arc A116 (39.1196, 22.2924) -> (39.7673, 20.8189) centre (41.1196, 22.2924) ccw projected
  line L63 (39.1196, 22.2924) -> (39.1196, 27.2485) projected
  arc A117 (39.7673, 28.7221) -> (39.1196, 27.2485) centre (41.1196, 27.2485) ccw projected
  arc A118 (39.937, 28.8646) -> (39.7673, 28.7221) centre (41.4696, 26.8672) ccw projected
  arc A119 (39.937, 28.8646) -> (40.7196, 30.4514) centre (38.7196, 30.4514) ccw projected
  line L64 (40.7196, 30.4514) -> (40.7196, 39.5896) projected
  arc A120 (40.7196, 39.5896) -> (39.937, 41.1764) centre (38.7196, 39.5896) ccw projected
  arc A121 (39.7673, 41.3189) -> (39.937, 41.1764) centre (41.4696, 43.1738) ccw projected
  arc A122 (39.1196, 42.7924) -> (39.7673, 41.3189) centre (41.1196, 42.7924) ccw projected
  line L65 (39.1196, 42.7924) -> (39.1196, 47.7485) projected
  arc A123 (39.7673, 49.2221) -> (39.1196, 47.7485) centre (41.1196, 47.7485) ccw projected
  arc A124 (43.3362, 49.0566) -> (39.7673, 49.2221) centre (41.4696, 47.3672) ccw projected
  arc A125 (43.3362, 49.0566) -> (44.819, 48.3987) centre (44.819, 50.3987) ccw projected
  line L66 (44.819, 48.3987) -> (75, 48.3987) projected
  line L67 (75, 48.3987) -> (75, 184.5) projected
  line L68 (75, 184.5) -> (57.5, 184.5) projected
  line L69 (57.5, 184.5) -> (57.5, 215) projected
  line L70 (57.5, 215) -> (-78, 215) projected
  line L71 (-78, 215) -> (-78, 46.0635) projected
  line L72 (-78, 46.0635) -> (-75, 46.0635) projected
  line L73 (-75, 46.0635) -> (-75, 40.8932) projected
  line L74 (-75, 40.8932) -> (-78, 40.8932) projected
  line L75 (-78, 40.8932) -> (-78, 30.6062) projected
  line L76 (-78, 30.6062) -> (-75, 30.6062) projected
  line L77 (-75, 30.6062) -> (-75, 20.5478) projected
  line L78 (-75, 20.5478) -> (-78, 20.5478) projected
  line L79 (-78, 20.5478) -> (-78, 10.2608) projected
  line L80 (-78, 10.2608) -> (-75, 10.2608) projected
  line L81 (-75, 10.2608) -> (-75, -0.1068) projected
  line L82 (-75, -0.1068) -> (-78, -0.1068) projected
  line L83 (-78, -0.1068) -> (-78, -10.3938) projected
  line L84 (-78, -10.3938) -> (-75, -10.3938) projected
  line L85 (-75, -10.3938) -> (-75, -20.4522) projected
  line L86 (-75, -20.4522) -> (-78, -20.4522) projected
  line L87 (-78, -20.4522) -> (-78, -30.7392) projected
  line L88 (-78, -30.7392) -> (-75, -30.7392) projected
  line L89 (-75, -30.7392) -> (-75, -41.1068) projected
  line L90 (-75, -41.1068) -> (-78, -41.1068) projected
  line L91 (-78, -41.1068) -> (-78, -51.3938) projected
  line L92 (-78, -51.3938) -> (-75, -51.3938) projected
  line L93 (-75, -51.3938) -> (-75, -61.4522) projected
  line L94 (-75, -61.4522) -> (-78, -61.4522) projected
  line L95 (-78, -61.4522) -> (-78, -71.7392) projected
  line L96 (-78, -71.7392) -> (-75, -71.7392) projected
  line L97 (-75, -71.7392) -> (-75, -82.1068) projected
  line L98 (-75, -82.1068) -> (-78, -82.1068) projected
  line L99 (-78, -82.1068) -> (-78, -92.3938) projected
  line L100 (-78, -92.3938) -> (-75, -92.3938) projected
  line L101 (-75, -92.3938) -> (-75, -102.4522) projected
  line L102 (-75, -102.4522) -> (-78, -102.4522) projected
  line L103 (-78, -102.4522) -> (-78, -112.7392) projected
  line L104 (-78, -112.7392) -> (-75, -112.7392) projected
  line L105 (-75, -112.7392) -> (-75, -130) projected
  line L106 (-75, -130) -> (-25.3933, -130) projected
  line L107 (-25.3933, -130) -> (-25.3933, -147.5) projected
  line L108 (-25.3933, -147.5) -> (23.6067, -147.5) projected
  line L109 (98, -130) -> (98, 184.5)
  line L110 (98, -130) -> (75, -130)
  line L111 (57.5, 215) -> (-78, 215) projected
  line L112 (80.4, 215) -> (57.5, 215)
  line L113 (98, 184.5) -> (80.4, 184.5)
  circle A126 centre (88, 174.5) radius 2.25
  circle A127 centre (88, 131.8987) radius 2.25
  circle A128 centre (88, 58.3987) radius 2.25
  circle A129 centre (88, -117.6237) radius 2.25
  line L114 (80.4, 184.5) -> (80.4, 215)
  arc A130 (64.4142, -110.1237) -> (63.7071, -110.4166) centre (64.4142, -111.1237) ccw projected
  line L115 (63.7071, -110.4166) -> (59.2929, -114.8308) projected
  line L116 (59.2929, -114.8308) -> (63.7071, -110.4166) projected
  arc A131 (63.7071, -110.4166) -> (64, -109.7094) centre (63, -109.7094) ccw
  line L117 (64, -109.7094) -> (64, -107.9669)
  line L118 (64, -107.9669) -> (64, 48.3987)
  line L119 (75, 48.3987) -> (44.819, 48.3987) projected
  circle A132 centre (65, -117.6237) radius 2.25
  circle A133 centre (65, 58.3987) radius 2.25
  circle A134 centre (65, 131.8987) radius 2.25
  circle A135 centre (65, 174.5) radius 2.25
  point P0 (0, 0)
  dimension "d46" = 176
  dimension "d47" = 4.5
  dimension "d48" = 10
  dimension "d49" = 4.5
  dimension "d50" = 10
  dimension "d51" = 4.5
  dimension "d52" = 10
  dimension "d53" = 4.5
  dimension "d54" = 10
  dimension "d55" = 17.6
  dimension "d57" = 1
  dimension "d66" = 2
  constraints: 15 end point, 9 centre point, 4 coincident, 4 concentric, 3 horizontal, 2 perpendicular, 2 point on circle, 2 tangent, 2 vertical, 1 point on line
  measures "d46" distance between parallel lines of L71 L109
  measures "d47" diameter of A126
  measures "d48" distance from line of L109 A126.centre
  measures "d49" diameter of A127
  measures "d50" distance from line of L109 A127.centre
  measures "d51" diameter of A128
  measures "d52" distance from line of L109 A128.centre
  measures "d53" diameter of A129
  measures "d54" distance from line of L109 A129.centre
  measures "d55" distance between parallel lines of L109 L114
  measures "d57" distance from line of L47 A75.centre
  measures "d66" diameter of A131
extrude "Extrusion6" add sketch "Sketch5" against normal blind 3 contours A8 | A9 | A10 | A11 | L46 A74 L47 A75 A131 L117 L118 L66 L67 L68 L69 L112 L114 L113 L109 L110